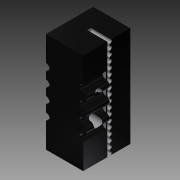
# Autodesk Inventor part: CueBeltHorder
Saved by Autodesk Inventor 2015 (Build 190159000, 159)
## iProperties
Created: 2017-01-09
Part Number: CueBeltHorder
Material: Generic
Document SubType Name: Modeling
Designer: Ernest
Density: 1 g/cm^3
Appearance: Default
Author: Ernest
Autodesk Inventor part; units mm, degrees
ref_plane "YZ Plane" through (0, 0, 0) normal (1, 0, 0) x (0, 1, 0)
ref_plane "XZ Plane" through (0, 0, 0) normal (0, 1, 0) x (-1, 0, 0)
ref_plane "XY Plane" through (0, 0, 0) normal (0, 0, 1) x (1, 0, 0)
sketch "Sketch1" plane through (0, 0, 0) normal (0, 0, 1) x (1, 0, 0)
  circle A0 centre (0, 0) radius 3
  circle A1 centre (51.029, 0) radius 3
  line L0 (-11, 0) -> (61.529, 0)
  circle A2 centre (0, 0) radius 6
  circle A3 centre (51.029, 0) radius 6
  line L1 (11, 0) -> (17.9507, 0)
  line L2 (33.0783, 0) -> (40.029, 0)
  line L3 (16.4475, -5) -> (16.4475, 0)
  line L4 (34.5815, -5) -> (34.5815, 0)
  line L5 (13.2571, 10) -> (13.2571, -10) construction
  line L6 (18.5272, 44.067) -> (39.0012, 44.067) construction
  line L7 (8.015, 33.5) -> (43.014, 33.5) construction
  line L8 (43.014, 33.5) -> (43.014, 15.5) construction
  line L9 (43.014, 15.5) -> (8.015, 15.5) construction
  line L10 (8.015, 15.5) -> (8.015, 33.5) construction
  line L11 (14.489, 24.5) -> (38.452, 24.5) construction
  line L12 (22.5145, 29) -> (28.5145, 29)
  line L13 (28.5145, 29) -> (28.5145, 20)
  line L14 (28.5145, 20) -> (22.5145, 20)
  line L15 (22.5145, 20) -> (22.5145, 29)
  line L16 (25.5145, 33.5) -> (25.5145, 15.5) construction
  line L17 (4.5826, 10) -> (46.4464, 10)
  line L18 (-13, 10) -> (-13, -10)
  line L19 (64.029, 10) -> (64.029, -10)
  line L20 (-13, 10) -> (-4.5826, 10)
  line L21 (-13, -10) -> (-4.5826, -10)
  line L22 (64.029, 10) -> (55.6116, 10)
  line L23 (64.029, -10) -> (55.6116, -10)
  line L24 (-11, 0) -> (-13, 0)
  line L25 (61.529, 0) -> (64.029, 0)
  arc A4 (11.8432, -9.8751) -> (39.1858, -9.8751) centre (25.5145, -5) ccw
  arc A5 (16.4475, -5) -> (34.5815, -5) centre (25.5145, -5) ccw
  arc A6 (33.0783, 0) -> (17.9507, 0) centre (25.5145, -5) ccw
  line L26 (46.1831, -9.8751) -> (39.1858, -9.8751)
  line L27 (4.8459, -9.8751) -> (11.8432, -9.8751)
  line L28 (11.2237, 0) -> (11.2238, -9.8751)
  line L29 (39.8053, 0) -> (39.8053, -9.8751)
  arc A7 (46.1831, -9.8751) -> (55.6116, -10) centre (51.029, 0) ccw
  arc A8 (55.6116, 10) -> (46.4464, 10) centre (51.029, 0) ccw
  arc A9 (4.5826, 10) -> (-4.5826, 10) centre (0, 0) ccw
  arc A10 (-4.5826, -10) -> (4.8459, -9.8751) centre (0, 0) ccw
  line L30 (6, 0) -> (6, -9.8751) construction
  line L31 (45.029, 0) -> (45.029, -9.8751) construction
  line L32 (30.5145, 26.5) -> (17.5145, 26.5)
  line L33 (17.5145, 26.5) -> (17.5145, 10)
  line L34 (17.5145, 10) -> (30.5145, 10)
  line L35 (30.5145, 10) -> (30.5145, 26.5)
  dimension "d4" = 12
  dimension "d5" = 12
  dimension "d0" = 6
  dimension "d1" = 6
  dimension "d2" = 51.029
  dimension "d8" = 20
  dimension "d9" = 10
  dimension "d11" = 15.5
  dimension "d12" = 33.5
  dimension "d13" = 8.015
  dimension "d14" = 8.015
  dimension "d15" = 9
  dimension "d16" = 9
  dimension "d17" = 4.5
  dimension "d18" = 6
  dimension "d19" = 34.999
  dimension "d21" = 3
  dimension "d23" = 2.5
  dimension "d24" = 20
  dimension "d25" = 10
  dimension "d26" = 20
  dimension "d27" = 10
  dimension "d28" = 25.5145
  dimension "d29" = 20.5
  dimension "d34" = 13
  dimension "d35" = 13
  dimension "d36" = 10.4475
  dimension "d37" = 10.4475
  dimension "d38" = 5.2237
  dimension "d39" = 5.2237
  dimension "d80" = 2
  dimension "d81" = 2
  dimension "d82" = 5
  constraints: 70 end point, 14 point on circle, 11 point on line, 9 centre point, 9 perpendicular, 8 horizontal, 7 parallel, 6 coincident, 5 vertical, 4 midpoint, 2 horizontal alignment, 2 tangent, 17 other
  measures "d0" diameter of A0
  measures "d1" diameter of A1
  measures "d2" distance of A1.centre point (0, 0)
  measures "d8" distance of L5.start L5.end
  measures "d9" distance from line of L1 L5.start
  measures "d11" distance from line of L9 point (0, 0)
  measures "d12" distance from line of L7 point (0, 0)
  measures "d13" distance from line of L10 point (0, 0)
  measures "d14" distance from line of L8 A1.centre
  measures "d15" distance between parallel lines of L9 L11
  measures "d16" distance of L14.end L12.start
  measures "d17" distance between parallel lines of L11 L12
  measures "d18" distance of L12.start L12.end
  measures "d19" distance of L7.start L7.end
  measures "d21" distance between parallel lines of L16 L13
  measures "d23" distance from line of L19 L25.start
  measures "d24" distance of L18.start L18.end
  measures "d25" vertical distance of L24.start L18.end
  measures "d26" distance of L19.start L19.end
  measures "d27" vertical distance of L25.start L19.end
  measures "d28" horizontal distance of A5.centre point (0, 0)
  measures "d29" distance from line of L9 A5.centre
  measures "d34" distance from line of point (0, 0) L18
  measures "d35" distance from line of L19 A1.centre
  measures "d36" distance between parallel lines of L3 L30
  measures "d37" distance between parallel lines of L31 L4
  measures "d38" distance between parallel lines of L28 L30
  measures "d39" distance between parallel lines of L29 L31
  measures "d80" distance between parallel lines of L13 L35
  measures "d81" distance between parallel lines of L11 L32
  measures "d82" distance between parallel lines of L15 L33
extrude "Extrusion1" add sketch "Sketch1" along normal blind 35 contours L0 A0 | A0 L0 A2 | A2 L0 L24 L18 L20 A9 L17 A8 L22 L19 L25 A3 A6 | L33 L32 L15 L14 L13 L35 L17 | L32 L13 L14 L15 | A3 L0 A1 | A1 L0 picked at (0.7485, 0.6631) picked at (3.2012, 3.7952) picked at (54.2302, 3.7952) picked at (51.5971, 1.7524)
extrude "Extrusion2" cut sketch "Sketch1" along normal blind 35 contours L0 A0 | L0 A2 A0 | A0 L0 A2 | A0 L0 | A3 L0 A1 | L0 A1 A3 | L0 A1 | A1 L0
sketch "Sketch2" plane through (-13, 0, 0) normal (0, -1, 0) x (1, 0, 0)
  line L0 (7, 0) -> (7, 35) projected
  line L1 (0, 35) -> (7, 35) projected
  line L2 (0, 0) -> (0, 35) projected
  line L3 (0, 0) -> (7, 0) projected
  line L4 (70.029, 35) -> (70.029, 0) projected
  line L5 (70.029, 0) -> (77.029, 0) projected
  line L6 (77.029, 0) -> (77.029, 35) projected
  line L7 (70.029, 35) -> (77.029, 35) projected
  line L8 (8.4174, 0) -> (0, 0) projected
  line L9 (0, 35) -> (1.157, 35)
  line L10 (1.157, 35) -> (1.157, 0)
  line L11 (1.157, 0) -> (0, 0)
  line L12 (0, 0) -> (0, 35)
  line L13 (70.029, 0) -> (77.029, 0) projected
  line L14 (77.029, 35) -> (75.872, 35)
  line L15 (75.872, 35) -> (75.872, 0)
  line L16 (75.872, 0) -> (77.029, 0)
  line L17 (77.029, 0) -> (77.029, 35)
  circle A0 centre (4.0785, 17.5) radius 1.5
  circle A1 centre (72.9505, 17.5) radius 1.5
  circle A2 centre (21.9215, 17.5) radius 1.5
  circle A3 centre (55.1075, 17.5) radius 1.5
  line L18 (19, 35) -> (19, 0) projected
  line L19 (19, 0) -> (30.9507, 0) projected
  line L20 (30.9507, 0) -> (30.9507, 35) projected
  line L21 (19, 35) -> (30.9507, 35) projected
  line L22 (58.029, 0) -> (58.029, 35) projected
  line L23 (46.0783, 35) -> (58.029, 35) projected
  line L24 (46.0783, 0) -> (46.0783, 35) projected
  line L25 (46.0783, 0) -> (58.029, 0) projected
  circle A4 centre (25.685, 29.167) radius 1.5
  circle A5 centre (25.685, 5.833) radius 1.5
  circle A6 centre (51.344, 29.167) radius 1.5
  circle A7 centre (51.344, 5.833) radius 1.5
  point P0 (13, 0)
  dimension "d44" = 11.843
  dimension "d45" = 1.157
  dimension "d46" = 1.157
  dimension "d50" = 3
  dimension "d52" = 3
  dimension "d53" = 5.843
  dimension "d54" = 2.9215
  dimension "d57" = 2.9215
  dimension "d58" = 35
  dimension "d59" = 17.5
  dimension "d60" = 17.5
  dimension "d61" = 3
  dimension "d62" = 3
  dimension "d63" = 17.5
  dimension "d64" = 17.5
  dimension "d65" = 2.9215
  dimension "d66" = 2.9215
  dimension "d67" = 3
  dimension "d68" = 3
  dimension "d69" = 3
  dimension "d70" = 3
  dimension "d71" = 5.833
  dimension "d72" = 5.833
  dimension "d73" = 5.833
  dimension "d74" = 5.833
  dimension "d75" = 6.685
  dimension "d76" = 6.685
  dimension "d77" = 6.685
  dimension "d78" = 6.685
  constraints: 16 end point, 8 centre point, 4 parallel, 2 horizontal, 2 perpendicular, 2 point on line
  measures "d44" distance from line of point (13, 0) L10
  measures "d45" distance between parallel lines of L2 L10
  measures "d46" distance between parallel lines of L6 L15
  measures "d50" diameter of A0
  measures "d52" diameter of A1
  measures "d53" distance between parallel lines of L0 L10
  measures "d54" distance from line of L0 A0.centre
  measures "d57" distance from line of L4 A1.centre
  measures "d58" distance of L0.start L0.end
  measures "d59" distance from line of L8 A0.centre
  measures "d60" distance from line of L5 A1.centre
  measures "d61" diameter of A2
  measures "d62" diameter of A3
  measures "d63" distance from line of L8 A2.centre
  measures "d64" distance from line of L13 A3.centre
  measures "d65" distance from line of L18 A2.centre
  measures "d66" distance from line of L22 A3.centre
  measures "d67" diameter of A4
  measures "d68" diameter of A5
  measures "d69" diameter of A6
  measures "d70" diameter of A7
  measures "d71" distance from line of L21 A4.centre
  measures "d72" distance from line of L19 A5.centre
  measures "d73" distance from line of L23 A6.centre
  measures "d74" distance from line of L25 A7.centre
  measures "d75" distance from line of L18 A4.centre
  measures "d76" distance from line of L18 A5.centre
  measures "d77" distance from line of L22 A6.centre
  measures "d78" distance from line of L22 A7.centre
extrude "Extrusion3" cut sketch "Sketch2" against normal blind 35 contours L3 L2 L1 L10 | L7 L6 L5 L15 | A0 | A1 | A2 | A3 | A4 | A5 | A6 | A7
sketch "Sketch3" plane through (30.5145, 10, 0) normal (1, 0, 0) x (0, 0, -1)
  line L0 (-35, 0) -> (-35, 16.5) projected
  line L1 (-35, 14.5) -> (0, 14.5) construction
  line L2 (0, 0) -> (0, 16.5) projected
  line L3 (0, 0) -> (0, 16.5) projected
  line L4 (0, 16.5) -> (-35, 16.5) projected
  line L5 (-35, 0) -> (-35, 16.5) projected
  line L6 (0, 0) -> (-35, 0) projected
  line L7 (-35, 19) -> (0, 19)
  line L8 (0, 19) -> (0, 10)
  line L9 (0, 10) -> (-35, 10)
  line L10 (-35, 10) -> (-35, 19)
  line L11 (-35, 10) -> (0, 10)
  line L12 (0, 10) -> (0, 8.4)
  line L13 (-32.5098, 8.4) -> (-34.5098, 8.4)
  line L14 (-35, 8.4) -> (-35, 10)
  arc A0 (-35, 9.054) -> (-35, 9.746) centre (-34.5098, 9.4) ccw
  circle A1 centre (-32.5098, 9.4) radius 0.6
  line L15 (-33.7098, 9.2) -> (-33.3098, 9.2)
  arc A2 (-33.9098, 9.4) -> (-33.7098, 9.2) centre (-33.7098, 9.4) ccw
  arc A3 (-33.3098, 9.2) -> (-33.1098, 9.4) centre (-33.3098, 9.4) ccw
  arc A4 (-35, 9.746) -> (-35, 9.054) centre (-34.5098, 9.4) ccw
  line L16 (-34.5098, 8.8) -> (-34.5098, 8.4)
  line L17 (-32.5098, 8.8) -> (-32.5098, 8.4)
  point P0 (0, -10)
  point P1 (-35, 9.2)
  point P2 (0, 9.2)
  point P3 (-33.9098, 9.4)
  point P4 (-33.1098, 9.4)
  dimension "d83" = 2
  dimension "d84" = 9
  dimension "d85" = 4.5
  dimension "d86" = 1.6
  dimension "d87" = 1.2
  dimension "d88" = 1.2
  dimension "d89" = 2
  dimension "d90" = 0.8
  dimension "d91" = 0.2
  constraints: 24 end point, 12 point on circle, 8 point on line, 5 centre point, 5 horizontal, 5 perpendicular, 4 parallel, 4 tangent, 2 coincident, 2 midpoint, 1 equal radius, 8 other
  measures "d83" distance between parallel lines of L1 L4
  measures "d84" distance between parallel lines of L9 L7
  measures "d85" distance between parallel lines of L1 L7
  measures "d86" distance between parallel lines of L11 L13
  measures "d87" diameter of A0
  measures "d88" diameter of A1
  measures "d89" distance of A1.centre A0.centre
  measures "d90" distance between parallel lines of L15 L13
  measures "d91" radius of A2
extrude "Extrusion4" cut sketch "Sketch3" against normal blind 7 contours L0 A0 | A0 A2 L15 A3 A1 L17 L13 L16 | A1
pattern_linear "Rectangular Pattern1" count 18 spacing 2 along (0, 0, -1) count 2 spacing 2 along (0, 0, 1) of "Extrusion4"
sketch "Sketch4" plane through (0, 0, 35) normal (0, 0, 1) x (1, 0, 0)
  line L0 (23.5145, 18.4) -> (23.5145, 19.746) projected
  line L1 (23.5145, 19.746) -> (30.5145, 19.746) projected
  line L2 (30.5145, 19.746) -> (30.5145, 26.5) projected
  line L3 (30.5145, 26.5) -> (17.5145, 26.5) projected
  line L4 (17.5145, 26.5) -> (17.5145, 10) projected
  line L5 (17.5145, 10) -> (4.5826, 10) projected
  arc A0 (4.5826, 10) -> (-4.5826, 10) centre (0, 0) ccw projected
  line L6 (-4.5826, 10) -> (-11.843, 10) projected
  line L7 (-11.843, 10) -> (-11.843, 0) projected
  line L8 (-11.843, 0) -> (-6, 0) projected
  arc A1 (6, 0) -> (-6, 0) centre (0, 0) ccw projected
  line L9 (6, 0) -> (17.9507, 0) projected
  arc A2 (33.0783, 0) -> (17.9507, 0) centre (25.5145, -5) ccw projected
  line L10 (33.0783, 0) -> (45.029, 0) projected
  arc A3 (57.029, 0) -> (45.029, 0) centre (51.029, 0) ccw projected
  line L11 (57.029, 0) -> (62.872, 0) projected
  line L12 (62.872, 0) -> (62.872, 10) projected
  line L13 (62.872, 10) -> (55.6116, 10) projected
  arc A4 (55.6116, 10) -> (46.4464, 10) centre (51.029, 0) ccw projected
  line L14 (46.4464, 10) -> (30.5145, 10) projected
  line L15 (30.5145, 10) -> (30.5145, 18.4) projected
  line L16 (30.5145, 18.4) -> (23.5145, 18.4) projected
  line L17 (17.5145, 10) -> (12.5145, 10)
  line L18 (12.5145, 10) -> (12.5145, 18)
  line L19 (12.5145, 18) -> (17.5145, 18)
  line L20 (17.5145, 18) -> (17.5145, 10)
  line L21 (30.5145, 10) -> (35.5145, 10)
  line L22 (35.5145, 10) -> (35.5145, 18)
  line L23 (35.5145, 18) -> (30.5145, 18)
  line L24 (30.5145, 18) -> (30.5145, 10)
  dimension "d100" = 8
  dimension "d101" = 5
  dimension "d106" = 5
  dimension "d107" = 8
  constraints: 16 end point, 4 parallel, 2 horizontal, 2 perpendicular
  measures "d100" distance of L17.end L18.end
  measures "d101" distance of L18.end L19.end
  measures "d106" distance of L23.end L22.end
  measures "d107" distance of L22.end L21.end
extrude "Extrusion5" add sketch "Sketch4" against normal blind 26.25 contours L23 L22 L14 L15 | L4 L5 L18 L19
extrude "Extrusion6" cut sketch "Sketch4" against normal blind 8.75 contours L23 L22 L14 L15 | L4 L5 L18 L19
sketch "Sketch5" plane through (17.5145, 26.5, 0) normal (0, 1, 0) x (1, 0, 0)
  arc A0 (0, -26.25) -> (0, -23.75) centre (0, -25) ccw
  line L0 (-5, -26.25) -> (0, -26.25) projected
  line L1 (-5, -8.75) -> (0, -8.75) projected
  arc A1 (0, -21.25) -> (0, -23.75) centre (0, -22.5) ccw
  arc A2 (0, -21.25) -> (0, -18.75) centre (0, -20) ccw
  arc A3 (0, -16.25) -> (0, -18.75) centre (0, -17.5) ccw
  arc A4 (0, -16.25) -> (0, -13.75) centre (0, -15) ccw
  arc A5 (0, -11.25) -> (0, -13.75) centre (0, -12.5) ccw
  arc A6 (0, -11.25) -> (0, -8.75) centre (0, -10) ccw
  arc A7 (13, -23.75) -> (13, -26.25) centre (13, -25) ccw
  line L2 (13, -26.25) -> (18, -26.25) projected
  arc A8 (13, -23.75) -> (13, -21.25) centre (13, -22.5) ccw
  arc A9 (13, -18.75) -> (13, -21.25) centre (13, -20) ccw
  arc A10 (13, -18.75) -> (13, -16.25) centre (13, -17.5) ccw
  arc A11 (13, -13.75) -> (13, -16.25) centre (13, -15) ccw
  arc A12 (13, -13.75) -> (13, -11.25) centre (13, -12.5) ccw
  arc A13 (13, -8.75) -> (13, -11.25) centre (13, -10) ccw
  line L3 (-29.291, -35) -> (0, -35)
  line L4 (0, 0) -> (-29.291, 0)
  line L5 (-29.291, 0) -> (-29.291, -35)
  line L6 (45.3575, -35) -> (13, -35)
  line L7 (13, 0) -> (45.3575, 0)
  line L8 (45.3575, 0) -> (45.3575, -35)
  line L9 (-5, -26.25) -> (0, -26.25)
  line L10 (0, -8.75) -> (-5, -8.75)
  line L11 (-5, -8.75) -> (-5, -26.25)
  line L12 (18, -26.25) -> (13, -26.25)
  line L13 (13, -8.75) -> (18, -8.75)
  line L14 (18, -8.75) -> (18, -26.25)
  line L15 (0, -8.75) -> (0, 0)
  line L16 (0, -35) -> (0, -26.25)
  line L17 (13, -35) -> (13, -26.25)
  line L18 (13, -8.75) -> (13, 0)
  line L19 (0, -35) -> (13, -35)
  line L20 (0, 0) -> (13, 0)
  point P0 (-17.5145, 0)
  dimension "d108" = 2.5
  dimension "d109" = 17.5
  dimension "d110" = 2.5
  dimension "d111" = 2.5
  dimension "d112" = 2.5
  dimension "d113" = 2.5
  dimension "d114" = 2.5
  dimension "d115" = 2.5
  dimension "d116" = 2.5
  dimension "d117" = 2.5
  dimension "d118" = 2.5
  dimension "d119" = 2.5
  dimension "d120" = 2.5
  dimension "d121" = 2.5
  dimension "d122" = 2.5
  constraints: 37 end point, 28 point on circle, 14 centre point, 13 tangent, 6 equal length, 5 horizontal, 1 point on line
  measures "d108" diameter of A0
  measures "d109" distance between parallel lines of L1 L0
  measures "d110" diameter of A1
  measures "d111" diameter of A2
  measures "d112" diameter of A3
  measures "d113" diameter of A4
  measures "d114" diameter of A5
  measures "d115" diameter of A6
  measures "d116" diameter of A7
  measures "d117" diameter of A8
  measures "d118" diameter of A9
  measures "d119" diameter of A10
  measures "d120" diameter of A11
  measures "d121" diameter of A12
  measures "d122" diameter of A13
extrude "Extrusion7" cut sketch "Sketch5" against normal blind 16.5 contours L0 L11 L1 A6 A5 A4 A3 A2 A1 A0 | A0 A1 A2 A3 A4 A5 A6 L15 L20 L18 A13 A12 A11 A10 A9 A8 A7 L17 L19 L16 | A7 A8 A9 A10 A11 A12 A13 L13 L14 L2 keep common part
extrude "Extrusion8" cut sketch "Sketch5" against normal up to surface (8 mm away) from surface at -8.5 contours L0 L11 L1 A6 A5 A4 A3 A2 A1 A0 | A7 A8 A9 A10 A11 A12 A13 L13 L14 L2
sketch "Sketch6" plane through (30.5145, 18.4, 35) normal (1, 0, 0) x (0, 0, -1)
  line L0 (26.25, -0.4) -> (26.25, -8.4) projected
  line L1 (35, -8.4) -> (26.25, -8.4) projected
  line L2 (35, -8.4) -> (35, 0) projected
  line L3 (35, 0) -> (0, 0) projected
  line L4 (0, -8.4) -> (0, 0) projected
  line L5 (0, -8.4) -> (8.75, -8.4) projected
  line L6 (8.75, -8.4) -> (8.75, -0.4) projected
  line L7 (8.75, -0.4) -> (11.25, -0.4) projected
  line L8 (11.25, -0.4) -> (13.75, -0.4) projected
  line L9 (13.75, -0.4) -> (16.25, -0.4) projected
  line L10 (16.25, -0.4) -> (18.75, -0.4) projected
  line L11 (18.75, -0.4) -> (21.25, -0.4) projected
  line L12 (21.25, -0.4) -> (23.75, -0.4) projected
  line L13 (23.75, -0.4) -> (26.25, -0.4) projected
  circle A0 centre (13.125, -4.4) radius 1.5
  circle A1 centre (21.875, -4.4) radius 1.5
  point P0 (35, -18.4)
  dimension "d127" = 8
  dimension "d128" = 17.5
  dimension "d129" = 3
  dimension "d130" = 3
  dimension "d131" = 4.375
  dimension "d132" = 4.375
  dimension "d133" = 4
  dimension "d134" = 4
  constraints: 2 centre point
  measures "d127" distance of L5.end L6.end
  measures "d128" distance between parallel lines of L6 L0
  measures "d129" diameter of A0
  measures "d130" diameter of A1
  measures "d131" distance from line of L6 A0.centre
  measures "d132" distance from line of L0 A1.centre
  measures "d133" distance from line of L8 A0.centre
  measures "d134" distance from line of L12 A1.centre
extrude "Extrusion9" cut sketch "Sketch6" along normal blind 2.75 and the other way blind 16.5 contours A0 | A1
sketch "Sketch7" plane through (17.5145, 26.5, 0) normal (0, 1, 0) x (1, 0, 0)
  line L0 (0, 0) -> (-2.1035, 0)
  line L1 (-2.1035, 0) -> (-2.1035, -35)
  line L2 (-2.1035, -35) -> (0, -35)
  line L3 (0, -35) -> (0, 0)
  point P0 (-17.5145, 0)
  constraints: 8 end point, 2 parallel, 1 horizontal, 1 perpendicular
extrude "Extrusion10" cut sketch "Sketch7" against normal blind 20.75
equation "\"d14\" = d13"
equation "\"d28\" = 0.5 * d2"
equation "\"d34\" = d35"
equation "\"d38\" = 0.5 * d36"
equation "\"d39\" = 0.5 * d37"
equation "\"d46\" = d45"
equation "\"d54\" = 0.5 * d53"
equation "\"d57\" = d54"
equation "\"d59\" = 0.5 * d58"
equation "\"d60\" = d59"
equation "\"d63\" = d59"
equation "\"d64\" = d60"
equation "\"d65\" = d57"
equation "\"d66\" = d57"
equation "\"d72\" = d71"
equation "\"d73\" = d71"
equation "\"d74\" = d72"
equation "\"d76\" = d75"
equation "\"d77\" = d75"
equation "\"d78\" = d75"
equation "\"d85\" = 0.5 * d84"
equation "\"d110\" = d108"
equation "\"d111\" = d108"
equation "\"d112\" = d108"
equation "\"d113\" = d108"
equation "\"d114\" = d108"
equation "\"d115\" = d108"
equation "\"d117\" = d116"
equation "\"d118\" = d116"
equation "\"d119\" = d116"
equation "\"d120\" = d116"
equation "\"d121\" = d116"
equation "\"d122\" = d116"
equation "\"d131\" = 0.25 * d128"
equation "\"d132\" = 0.25 * d128"
equation "\"d133\" = 0.5 * d127"
equation "\"d134\" = d133"
body "Solid1"
